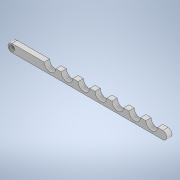
# Autodesk Inventor part: u_grosse_Hoehenverstellung
Saved by Autodesk Inventor 2020.3 (Build 243373000, 373)
## iProperties
Created: 2020-10-04
Part Number: u_grosse_Hoehenverstellung
Material: Generic
Document SubType Name: Modeling
Designer: Mara
Density: 1 g/cm^3
Appearance: Default
Author: Mara
Autodesk Inventor part; units mm, degrees
ref_plane "YZ Plane" through (0, 0, 0) normal (1, 0, 0) x (0, 1, 0)
ref_plane "XZ Plane" through (0, 0, 0) normal (0, 1, 0) x (-1, 0, 0)
ref_plane "XY Plane" through (0, 0, 0) normal (0, 0, 1) x (1, 0, 0)
sketch "Sketch1" plane through (0, 0, 0) normal (0, 0, 1) x (1, 0, 0)
  line L0 (-285, -15) -> (285, -15)
  line L1 (285, -15) -> (285, 15) construction
  line L2 (285, 15) -> (-285, 15)
  line L3 (-285, 15) -> (-285, -15) construction
  line L4 (-285, -15) -> (285, 15) construction
  line L5 (285, -15) -> (-285, 15) construction
  arc A0 (-285, 15) -> (-285, -15) centre (-285, 0) ccw
  arc A1 (285, -15) -> (285, 15) centre (285, 0) ccw
  point P0 (0, 0)
  dimension "d0" = 570
  dimension "d1" = 30
  constraints: 12 end point, 4 midpoint, 4 point on circle, 2 centre point, 2 parallel, 1 horizontal, 1 perpendicular
  measures "d0" distance of L2.end L1.end
  measures "d1" distance of L1.end L0.end
extrude "Extrusion1" add sketch "Sketch1" along normal blind 20
sketch "Sketch2" plane through (0, 0, 20) normal (0, 0, 1) x (1, 0, 0)
  arc A0 (-285, 15) -> (-285, -15) centre (-285, 0) ccw projected
  circle A1 centre (-285, 0) radius 10
  point P0 (0, 0)
  dimension "d4" = 20
  constraints: 1 centre point, 1 coincident
  measures "d4" diameter of A1
extrude "Extrusion2" cut sketch "Sketch2" against normal blind 15
sketch "Sketch3" plane through (0, 0, 20) normal (0, 0, 1) x (1, 0, 0)
  line L0 (285, 15) -> (-285, 15) projected
  arc A0 (221, 15) -> (265, 15) centre (243, 15) ccw
  arc A1 (157, 15) -> (201, 15) centre (179, 15) ccw
  arc A2 (93, 15) -> (137, 15) centre (115, 15) ccw
  arc A3 (29, 15) -> (73, 15) centre (51, 15) ccw
  arc A4 (-35, 15) -> (9, 15) centre (-13, 15) ccw
  arc A5 (-99, 15) -> (-55, 15) centre (-77, 15) ccw
  arc A6 (-163, 15) -> (-119, 15) centre (-141, 15) ccw
  point P0 (0, 0)
  dimension "d8" = 20
  dimension "d9" = 22
  dimension "d10" = 22
  dimension "d11" = 64
  dimension "d12" = 22
  dimension "d13" = 22
  dimension "d14" = 64
  dimension "d15" = 64
  dimension "d16" = 22
  dimension "d17" = 64
  dimension "d18" = 22
  dimension "d19" = 22
  dimension "d20" = 64
  dimension "d21" = 64
  constraints: 14 point on circle, 7 centre point, 22 other
  measures "d8" distance of A0.end point (285, 15)
  measures "d9" radius of A0
  measures "d10" radius of A1
  measures "d11" distance of A0.centre A1.centre
  measures "d12" radius of A2
  measures "d13" radius of A3
  measures "d14" distance of A1.centre A2.centre
  measures "d15" distance of A2.centre A3.centre
  measures "d16" radius of A4
  measures "d17" distance of A3.centre A4.centre
  measures "d18" radius of A5
  measures "d19" radius of A6
  measures "d20" distance of A5.centre A4.centre
  measures "d21" distance of A6.centre A5.centre
extrude "Extrusion3" cut sketch "Sketch3" against normal through all
equation "\"d10\" = d9"
equation "\"d11\" = d8 + 2 * d9"
equation "\"d12\" = d9"
equation "\"d13\" = d9"
equation "\"d14\" = d11"
equation "\"d15\" = d11"
equation "\"d16\" = d9"
equation "\"d17\" = d11"
equation "\"d18\" = d9"
equation "\"d19\" = d9"
equation "\"d20\" = d11"
equation "\"d21\" = d11"
body "Solid1"
